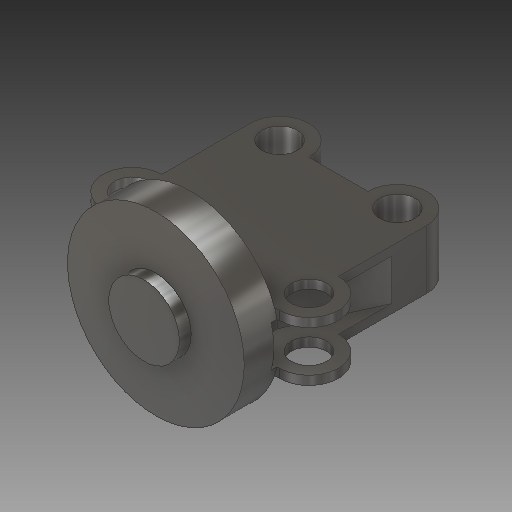
# Autodesk Inventor part: Pam
Saved by Autodesk Inventor 2019 (Build 230136000, 136)
## iProperties
Created: 2018-12-28
Part Number: Pam
Material: 钢，高强度，低合金
Document SubType Name: Modeling
Designer: JianQiao Hu
Density: 7.85 g/cm^3
Appearance: 钢 - 抛光
Author: JianQiao Hu
Autodesk Inventor part; units mm, degrees
ref_plane "YZ Plane" through (0, 0, 0) normal (1, 0, 0) x (0, 1, 0)
ref_plane "XZ Plane" through (0, 0, 0) normal (0, 1, 0) x (-1, 0, 0)
ref_plane "XY Plane" through (0, 0, 0) normal (0, 0, 1) x (1, 0, 0)
sketch "草图1" plane through (0, 0, 0) normal (0, 0, 1) x (1, 0, 0)
  circle A0 centre (0, 0) radius 75
  dimension "d0" = 150
  constraints: 1 centre point, 1 coincident
  measures "d0" diameter of A0
extrude "拉伸1" add sketch "草图1" along normal blind 30
sketch "草图2" plane through (0, 0, 30) normal (0, 0, 1) x (1, 0, 0)
  circle A0 centre (0, 0) radius 30
  dimension "d3" = 60
  constraints: 1 centre point, 1 coincident
  measures "d3" diameter of A0
extrude "拉伸2" add sketch "草图2" along normal blind 10
sketch "草图3" plane through (0, 0, 0) normal (0, 0, -1) x (-1, 0, 0)
  circle A0 centre (0, 0) radius 75 projected
  line L0 (-75, 25) -> (75, 25)
  line L1 (75, 25) -> (75, -25)
  line L2 (75, -25) -> (-75, -25)
  line L3 (-75, -25) -> (-75, 25)
  line L4 (-75, 25) -> (75, -25) construction
  line L5 (75, 25) -> (-75, -25) construction
  dimension "d21" = 50
  dimension "d22" = 150
  constraints: 12 end point, 2 midpoint, 2 parallel, 1 horizontal, 1 perpendicular
  measures "d21" distance of L0.end L1.end
  measures "d22" distance of L1.end L2.end
extrude "拉伸3" add sketch "草图3" along normal blind 150 contours A0 L2 L0 | L1 L2 A0 | A0 L0 L1 | A0 L3 L0 | L2 L3 A0
sketch "草图4" plane through (-70, 25, 0) normal (0, 1, 0) x (1, 0, 0)
  circle A0 centre (120, 125) radius 15
  circle A1 centre (20, 125) radius 15
  line L0 (145, 0) -> (145, 150) projected
  arc A2 (145, 125) -> (95, 125) centre (120, 125) ccw
  line L1 (-5, 150) -> (145, 150) projected
  arc A3 (45, 125) -> (-5, 125) centre (20, 125) ccw
  line L2 (145, 125) -> (145, 150)
  line L3 (120, 150) -> (20, 150)
  line L4 (-5, 0) -> (-5, 150) projected
  line L5 (-5, 150) -> (20, 150)
  line L6 (-5, 150) -> (-5, 125)
  line L7 (95, 125) -> (45, 125)
  point P0 (70, 0)
  dimension "d12" = 30
  dimension "d13" = 30
  dimension "d23" = 100
  dimension "d24" = 25
  constraints: 10 end point, 6 point on circle, 4 centre point, 4 tangent, 3 point on line, 2 coincident, 2 collinear, 1 perpendicular
  measures "d12" diameter of A0
  measures "d13" diameter of A1
  measures "d23" distance of A1.centre A0.centre
  measures "d24" distance from line of L0 A0.centre
extrude "拉伸4" cut sketch "草图4" against normal through all
sketch "草图5" plane through (-70.7107, -25, 0) normal (0, -1, 0) x (1, 0, 0)
  line L0 (-4.2893, 0) -> (-4.2893, -125) projected
  line L1 (145.7107, 0) -> (145.7107, -125) projected
  line L2 (0, 0) -> (141.4214, 0) projected
  circle A0 centre (-4.2893, -25) radius 25
  circle A1 centre (145.7107, -25) radius 25
  circle A2 centre (-4.2893, -25) radius 15
  circle A3 centre (145.7107, -25) radius 15
  point P0 (70.7107, 0)
  dimension "d34" = 30
  dimension "d35" = 30
  constraints: 2 centre point, 2 coincident, 2 vertical alignment, 4 other
  measures "d34" diameter of A2
  measures "d35" diameter of A3
extrude "拉伸5" add sketch "草图5" against normal up to surface (50 mm away) contours A0 L0 A2 | L0 A2 A0 | A1 L1 A3 | L1 A3 A1
extrude "拉伸6" cut sketch "草图5" against normal through all contours A2 L0 | L0 A2 | A3 L1 | L1 A3
sketch "草图6" plane through (0, 0, 0) normal (0, 1, 0) x (-1, 0, 0)
  circle A0 centre (75, -25) radius 15 projected
  circle A1 centre (75, -25) radius 30
  circle A2 centre (-75, -25) radius 15 projected
  circle A3 centre (-75, -25) radius 30
  point P0 (0, 0)
  dimension "d40" = 60
  dimension "d41" = 60
  constraints: 2 centre point, 2 coincident
  measures "d40" diameter of A3
  measures "d41" diameter of A1
extrude "拉伸7" cut sketch "草图6" along normal mid plane 35
chamfer "倒角1" distance 40 angle 45 2 edges at (-75, 0, -55) (75, 0, -55)
equation "\"d36\" = d13"
equation "\"d38\" = d13"
